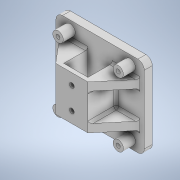
# Autodesk Inventor part: щустрик 1 model 2
Saved by Autodesk Inventor 2022.2 (Build 262287010, 287A)
## iProperties
Created: 2023-12-28
Part Number: щустрик 1 model 2
Material: Типовые
Document SubType Name: Modeling
Designer: 102-4
Density: 1 g/cm^3
Appearance: По умолчанию
Author: 102-4
## iProperties of the stored document щустрик 1 model 2_3DПЕЧАТЬ.ipt
Created: 2023-12-28
Part Number: щустрик 1 model 2_3DПЕЧАТЬ
Material: Типовые
Document SubType Name: Modeling
Designer: 102-4
Density: 1 g/cm^3
Appearance: По умолчанию
Author: 102-4
Autodesk Inventor part; units mm, degrees
ref_plane "YZ Plane" through (0, 0, 0) normal (1, 0, 0) x (0, 1, 0)
ref_plane "XZ Plane" through (0, 0, 0) normal (0, 1, 0) x (-1, 0, 0)
ref_plane "XY Plane" through (0, 0, 0) normal (0, 0, 1) x (1, 0, 0)
sketch "Эскиз1" plane through (0, 0, 0) normal (0, 0, 1) x (1, 0, 0)
  line L0 (0, 0) -> (-110, 0)
  line L1 (-110, 0) -> (-110, 135)
  line L2 (-110, 135) -> (0, 135)
  line L3 (0, 135) -> (0, 0)
  dimension "d0" = 135
  dimension "d1" = 110
  constraints: 8 end point, 2 parallel, 1 coincident, 1 horizontal, 1 perpendicular
  measures "d0" distance of L2.end L0.start
  measures "d1" distance between parallel lines of L1 L3
extrude "Выдавливание1" add sketch "Эскиз1" along normal blind 10
sketch "Эскиз2" plane through (0, 0, 10) normal (0, 0, 1) x (1, 0, 0)
  line L0 (-110, 37.5) -> (-110, 97.5)
  line L1 (0, 97.5) -> (0, 37.5)
  line L2 (0, 135) -> (-110, 135) projected
  line L3 (-110, 135) -> (-110, 0) projected
  line L4 (-110, 135) -> (-110, 0)
  line L5 (-92.55, 0) -> (-92.55, 37.5)
  line L6 (-17.45, 37.5) -> (-17.45, 39.5)
  line L7 (-17.45, 39.5) -> (-17.45, 15.5)
  circle A0 centre (-17.45, 27.5) radius 2.55
  line L8 (-55, 0) -> (-55, 135)
  line L9 (0, 0) -> (0, 135) projected
  line L10 (0, 67.5) -> (-110, 67.5)
  circle A1 centre (-17.45, 107.5) radius 2.55
  circle A2 centre (-92.45, 27.5) radius 2.55
  circle A3 centre (-92.45, 107.5) radius 2.55
  line L11 (-70.1, 92.5) -> (-39.9, 92.5)
  line L12 (-39.9, 92.5) -> (-39.9, 42.5)
  line L13 (-70.1, 42.5) -> (-70.1, 92.5)
  line L14 (-70.1, 92.5) -> (-39.9, 42.5) construction
  line L15 (-39.9, 92.5) -> (-70.1, 42.5) construction
  line L16 (-34.9, 97.5) -> (-75.1, 97.5)
  line L17 (-39.9, 42.5) -> (-34.9, 42.5)
  line L18 (-34.9, 42.5) -> (-34.9, 97.5)
  line L19 (-70.1, 42.5) -> (-75.1, 42.5)
  line L20 (-75.1, 42.5) -> (-75.1, 97.5)
  point P0 (-55, 67.5)
  dimension "d11" = 24
  dimension "d12" = 5.1
  dimension "d15" = 80
  dimension "d18" = 75
  dimension "d48" = 30.2
  constraints: 36 end point, 9 midpoint, 4 centre point, 3 equal length, 3 perpendicular, 2 coincident, 2 horizontal, 1 point on line, 1 vertical, 6 other
  measures "d11" distance of L6.end L7.end
  measures "d12" diameter of A0
  measures "d15" distance of A0.centre A1.centre
  measures "d18" distance of A0.centre A2.centre
  measures "d48" distance between parallel lines of L13 L12
extrude "Выдавливание2" cut sketch "Эскиз2" against normal through all contours A2 L5 | L5 A2 | A0 L7 | L7 A0 | A1 | A3
extrude "Выдавливание3" add sketch "Эскиз2" along normal blind 30.2 contours L20 L16 L8 L11 L13 L10 | L10 L13 L19 L20 | L16 L18 L10 L12 L11 L8 | L10 L18 L17 L12
sketch "Эскиз3" plane through (0, 0, 40.2) normal (0, 0, 1) x (1, 0, 0)
  line L0 (-75.1, 97.5) -> (-34.9, 97.5) projected
  line L1 (-75.1, 42.5) -> (-75.1, 97.5) projected
  line L2 (-34.9, 97.5) -> (-75.1, 97.5)
  line L3 (-75.1, 97.5) -> (-75.1, 42.5)
  line L4 (-75.1, 42.5) -> (-34.9, 42.5)
  line L5 (-34.9, 42.5) -> (-34.9, 97.5)
  point P0 (0, 0)
  constraints: 8 end point, 2 parallel, 1 horizontal, 1 perpendicular
extrude "Выдавливание4" add sketch "Эскиз3" along normal blind 5
ref_plane "РабПлоскость5" through (-110, 10, 0) normal (0, -1, 0) x (1, 0, 0)
sketch "Эскиз11" plane through (0, 0, 0) normal (0, 0, -1) x (-1, 0, 0)
  line L0 (110, 135) -> (110, 0) projected
  line L1 (110, 135) -> (0, 135)
  line L2 (0, 135) -> (0, 0)
  line L3 (0, 0) -> (110, 0)
  line L4 (110, 0) -> (110, 135)
  line L5 (3.3, 131.7) -> (106.7, 131.7)
  line L6 (106.7, 131.7) -> (106.7, 3.3)
  line L7 (106.7, 3.3) -> (3.3, 3.3)
  line L8 (3.3, 3.3) -> (3.3, 131.7)
  line L9 (110, 37.5) -> (110, 97.5)
  line L10 (0, 0) -> (0, 135) projected
  line L11 (0, 97.5) -> (110, 97.5)
  line L12 (110, 97.5) -> (110, 37.5)
  line L13 (110, 37.5) -> (0, 37.5)
  line L14 (0, 37.5) -> (0, 97.5)
  line L15 (106.7, 97.5) -> (106.7, 135)
  line L16 (3.3, 97.5) -> (3.3, 135)
  line L17 (0, 135) -> (110, 135) projected
  line L18 (3.3, 37.5) -> (3.3, 0)
  line L19 (110, 0) -> (0, 0) projected
  line L20 (106.7, 37.5) -> (106.7, 0)
  point P0 (3.3, 67.5)
  point P1 (3.3, 0)
  point P2 (3.3, 3.3)
  point P3 (0, 37.5)
  point P4 (106.7, 3.3)
  point P5 (106.7, 0)
  point P6 (106.7, 131.7)
  dimension "d42" = 3.3
  constraints: 34 end point, 16 point on line, 7 parallel, 3 perpendicular, 2 horizontal, 1 midpoint, 3 other
  measures "d42" distance between parallel lines of L1 L5
extrude "Выдавливание7" add sketch "Эскиз11" along normal blind 31 contours L0 L11 L6 L15 L1 | L0 L3 L20 L6 L13 | L16 L8 L11 L2 L1 | L8 L18 L3 L2 L13
sketch "Эскиз12" plane through (0, 0, -31) normal (0, 0, -1) x (-1, 0, 0)
  line L0 (110, 135) -> (110, 0) projected
  line L1 (0, 0) -> (0, 135) projected
  line L2 (110, 135) -> (0, 135)
  line L3 (0, 135) -> (0, 0)
  line L4 (0, 0) -> (110, 0)
  line L5 (110, 0) -> (110, 135)
  constraints: 8 end point, 2 parallel, 1 horizontal, 1 perpendicular
extrude "Выдавливание8" add sketch "Эскиз12" along normal blind 5
sketch "Эскиз13" plane through (0, 0, 45.2) normal (0, 0, 1) x (1, 0, 0)
  line L0 (-75.1, 97.5) -> (-34.9, 97.5) projected
  line L1 (-55, 97.5) -> (-55, 42.5)
  line L2 (-70.1, 42.5) -> (-39.9, 42.5) projected
  line L3 (-55, 70) -> (-55, 97.5)
  line L4 (-55, 70) -> (-55, 42.5)
  circle A0 centre (-55, 83.75) radius 3
  circle A1 centre (-55, 56.25) radius 3
  point P0 (0, 0)
  point P1 (-75.1, 42.5)
  dimension "d77" = 6
  dimension "d78" = 6
  constraints: 6 end point, 5 midpoint, 2 centre point, 2 collinear
  measures "d77" diameter of A0
  measures "d78" diameter of A1
extrude "Выдавливание9" cut sketch "Эскиз13" against normal blind 10
sketch "Эскиз14" plane through (-110, 0, 10) normal (-1, 0, 0) x (0, 0, 1)
  line L0 (-24.5, 100) -> (-24.5, 95)
  line L1 (-24.5, 95) -> (-26.5, 95)
  line L2 (-26.5, 95) -> (-26.5, 100)
  line L3 (-26.5, 100) -> (-24.5, 100)
  line L4 (-10, 97.5) -> (-41, 97.5) projected
  line L5 (-24.5, 100) -> (-26.5, 95) construction
  line L6 (-24.5, 95) -> (-26.5, 100) construction
  line L7 (-20.4, 100) -> (-30.6, 100)
  line L8 (-30.6, 100) -> (-30.6, 101.5)
  line L9 (-30.6, 101.5) -> (-20.4, 101.5)
  line L10 (-20.4, 101.5) -> (-20.4, 100)
  line L11 (-10, 97.5) -> (-10, 37.5) projected
  line L12 (-10, 67.5) -> (-41, 67.5)
  line L13 (-41, 97.5) -> (-41, 37.5) projected
  line L14 (-20.4, 35) -> (-30.6, 35)
  line L15 (-30.6, 35) -> (-30.6, 33.5)
  line L16 (-30.6, 33.5) -> (-20.4, 33.5)
  line L17 (-20.4, 33.5) -> (-20.4, 35)
  point P0 (-10, 0)
  point P1 (-25.5, 97.5)
  point P2 (-25.5, 100)
  dimension "d55" = 5
  dimension "d56" = 2
  dimension "d57" = 10.2
  dimension "d58" = 1.5
  constraints: 30 end point, 7 midpoint, 4 parallel, 4 symmetric about line, 2 perpendicular, 1 horizontal, 1 vertical
  measures "d55" distance of L0.start L0.end
  measures "d56" distance between parallel lines of L2 L0
  measures "d57" distance of L8.end L9.end
  measures "d58" distance of L7.end L8.end
extrude "Выдавливание10" cut sketch "Эскиз14" against normal through all contours L0 L4 L2 L3 | L3 L7 L8 L9 L10 | L0 L1 L2 L4
extrude "Выдавливание11" cut sketch "Эскиз14" against normal through all contours L17 L16 L15 L14
sketch "Эскиз15" plane through (-39.9, 42.5, 10) normal (0, -1, 0) x (1, 0, 0)
  line L0 (-35.2, 35.2) -> (5, 35.2) projected
  line L1 (-35.2, 35.2) -> (-64.7363, 0)
  line L2 (-70.1, 0) -> (39.9, 0) projected
  line L3 (-35.2, 35.2) -> (10.7503, 35.2) construction
  line L4 (-64.7363, 0) -> (-35.2, 0)
  line L5 (-35.2, 35.2) -> (-35.2, 0)
  line L6 (-35.2, 35.2) -> (5, 35.2)
  line L7 (5, 35.2) -> (-15.1, 35.2)
  line L8 (-15.1, 35.2) -> (-15.1, 0)
  line L9 (-64.7363, 0) -> (-35.2, 0)
  line L10 (5, 35.2) -> (34.5363, 0)
  line L11 (5, 35.2) -> (5, 0)
  line L12 (5, 0) -> (34.5363, 0)
  point P0 (39.9, -10)
  dimension "d63" = 130
  constraints: 22 end point, 3 point on line, 2 collinear, 2 perpendicular, 2 symmetric about line, 1 equal length, 1 horizontal, 1 midpoint
  measures "d63" angle of L1 L3
extrude "Выдавливание12" add sketch "Эскиз15" against normal blind 10 contours L5 L2 L1 | L10 L2 L11
sketch "Эскиз16" plane through (0, 0, 0) normal (0, 0, -1) x (-1, 0, 0)
  line L0 (-81.5108, 199.1539) -> (168.849, 199.1539)
  line L1 (168.849, 199.1539) -> (168.849, -122.7373)
  line L2 (168.849, -122.7373) -> (-81.5108, -122.7373)
  line L3 (-81.5108, -122.7373) -> (-81.5108, 199.1539)
  point P0 (0, 0)
  constraints: 8 end point, 2 parallel, 1 horizontal, 1 perpendicular
extrude "Выдавливание13" cut sketch "Эскиз16" along normal blind 42.75
delete faces "Удаление грани1" heal yes whole lump no faces at (-60.0333, 92.5, 20.0667)
ref_plane "РабПлоскость6" through (-75.1, 70, 45.2) normal (0, 1, 0) x (1, 0, 0)
mirror "Зеркальное отражение1" about plane through (-75.1, 70, 45.2) normal (0, 1, 0) of "Выдавливание12"
fillet "Сопряжение1" radius 3 4 edges at (-75.1, 52.5, 27.6) (-75.1, 87.5, 27.6) (-34.9, 87.5, 27.6) (-34.9, 52.5, 27.6)
fillet "Сопряжение2" radius 3 14 edges at (-75.9787, 86.6213, 10) (-91.3682, 87.5, 10) (-75.9787, 53.3787, 10) (-91.3682, 52.5, 10) (-75.1, 70, 10) (-34.0213, 53.3787, 10) (-18.6318, 52.5, 10) (-34.0213, 86.6213, 10) (-18.6318, 87.5, 10) (-34.9, 70, 10) (-22.6318, 42.5, 10) (-87.3682, 42.5, 10) (-87.3682, 97.5, 10) (-22.6318, 97.5, 10)
fillet "Сопряжение3" radius 8 4 edges at (0, 0, 5) (-110, 0, 5) (0, 135, 5) (-110, 135, 5)
move faces "Перенос1" translate (0, 17, 0) faces at (-70.6667, 0, 3.3333)
move faces "Перенос2" translate (0, -17, 0) faces at (-60.0333, 135, 6.6667)
sketch "Эскиз17" plane through (-110, 25, 10) normal (0, 0, 1) x (1, 0, 0)
  circle A0 centre (92.55, 82.5) radius 2.55 projected
  circle A1 centre (92.55, 82.5) radius 6.5
  line L0 (110, 0) -> (110, 85) projected
  line L1 (110, 42.5) -> (0, 42.5)
  line L2 (0, 85) -> (0, 0) projected
  line L3 (102, 93) -> (8, 93) projected
  line L4 (55, 93) -> (55, -8)
  line L5 (8, -8) -> (102, -8) projected
  circle A2 centre (17.55, 82.5) radius 6.5
  circle A3 centre (92.55, 2.5) radius 6.5
  circle A4 centre (17.55, 2.5) radius 6.5
  circle A5 centre (92.55, 82.5) radius 2.55
  circle A6 centre (17.55, 82.5) radius 2.55
  circle A7 centre (92.55, 2.5) radius 2.55
  circle A8 centre (17.55, 2.5) radius 2.55
  point P0 (110, -25)
  point P1 (94.283, 80.6294)
  dimension "d79" = 13
  dimension "d82" = 75
  dimension "d85" = 80
  dimension "d90" = 75
  dimension "d93" = 80
  constraints: 8 centre point, 4 end point, 4 midpoint, 3 coincident, 2 horizontal, 2 vertical, 15 other
  measures "d79" diameter of A1
  measures "d82" distance of A1.centre A2.centre
  measures "d85" distance of A1.centre A3.centre
  measures "d90" distance of A5.centre A6.centre
  measures "d93" distance of A5.centre A7.centre
extrude "Выдавливание14" add sketch "Эскиз17" along normal blind 15
